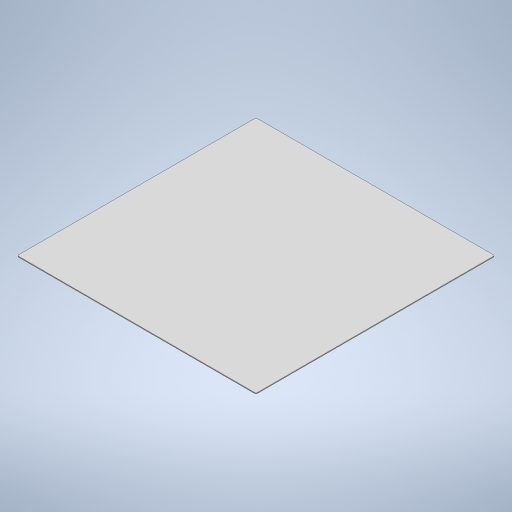
# Autodesk Inventor part: Glass top X1
Saved by Autodesk Inventor 2023 (Build 270158000, 158)
## iProperties
Created: 2022-11-22
Part Number: Glass top X1
Material: Generic
Document SubType Name: Modeling
Designer: surat
Density: 1 g/cm^3
Appearance: Default
Author: surat
Autodesk Inventor part; units mm, degrees
ref_plane "YZ Plane" through (0, 0, 0) normal (1, 0, 0) x (0, 1, 0)
ref_plane "XZ Plane" through (0, 0, 0) normal (0, 1, 0) x (-1, 0, 0)
ref_plane "XY Plane" through (0, 0, 0) normal (0, 0, 1) x (1, 0, 0)
sketch "Sketch1" plane through (0, 0, 0) normal (0, 1, 0) x (-1, 0, 0)
  line L0 (6.35, 0) -> (1365.25, 0)
  line L1 (1371.6, -6.35) -> (1371.6, -1365.25)
  line L2 (1365.25, -1371.6) -> (6.35, -1371.6)
  line L3 (0, -1365.25) -> (0, -6.35)
  line L4 (1346.2, -1346.2) -> (1346.2, -25.4)
  line L5 (1346.2, -25.4) -> (25.4, -25.4)
  line L6 (25.4, -25.4) -> (25.4, -1346.2)
  line L7 (25.4, -1346.2) -> (1346.2, -1346.2)
  line L8 (1320.8, -50.8) -> (1320.8, -1320.8)
  line L9 (1320.8, -1320.8) -> (50.8, -1320.8)
  line L10 (50.8, -1320.8) -> (50.8, -50.8)
  line L11 (50.8, -50.8) -> (1320.8, -50.8)
  line L12 (1320.8, -50.8) -> (1346.2, -25.4)
  line L13 (1320.8, -1320.8) -> (1346.2, -1346.2)
  line L14 (50.8, -1320.8) -> (25.4, -1346.2)
  line L15 (50.8, -50.8) -> (25.4, -25.4)
  line L16 (1219.2, -482.6) -> (1016, -482.6)
  line L17 (1016, -482.6) -> (1016, -889)
  line L18 (1016, -889) -> (1219.2, -889)
  line L19 (1219.2, -889) -> (1219.2, -482.6)
  line L20 (355.6, -482.6) -> (152.4, -482.6)
  line L21 (152.4, -482.6) -> (152.4, -889)
  line L22 (152.4, -889) -> (355.6, -889)
  line L23 (355.6, -889) -> (355.6, -482.6)
  line L24 (889, -1016) -> (482.6, -1016)
  line L25 (482.6, -1016) -> (482.6, -1219.2)
  line L26 (482.6, -1219.2) -> (889, -1219.2)
  line L27 (889, -1219.2) -> (889, -1016)
  line L28 (889, -152.4) -> (482.6, -152.4)
  line L29 (482.6, -152.4) -> (482.6, -355.6)
  line L30 (482.6, -355.6) -> (889, -355.6)
  line L31 (889, -355.6) -> (889, -152.4)
  circle A0 centre (685.8, -685.8) radius 254
  line L32 (889, -127) -> (482.6, -127)
  line L33 (457.2, -127) -> (457.2, -381)
  line L34 (457.2, -381) -> (914.4, -381)
  line L35 (914.4, -381) -> (914.4, -127)
  line L36 (1244.6, -457.2) -> (990.6, -457.2)
  line L37 (990.6, -457.2) -> (990.6, -914.4)
  line L38 (990.6, -914.4) -> (1244.6, -914.4)
  line L39 (1244.6, -889) -> (1244.6, -482.6)
  line L40 (914.4, -990.6) -> (457.2, -990.6)
  line L41 (457.2, -990.6) -> (457.2, -1244.6)
  line L42 (482.6, -1244.6) -> (889, -1244.6)
  line L43 (914.4, -1244.6) -> (914.4, -990.6)
  line L44 (381, -457.2) -> (127, -457.2)
  line L45 (127, -482.6) -> (127, -889)
  line L46 (127, -914.4) -> (381, -914.4)
  line L47 (381, -914.4) -> (381, -457.2)
  line L48 (152.4, -482.6) -> (50.8, -482.6)
  line L49 (127, -457.2) -> (50.8, -457.2)
  line L50 (152.4, -889) -> (50.8, -889)
  line L51 (127, -914.4) -> (50.8, -914.4)
  line L52 (355.6, -889) -> (381, -889)
  line L53 (355.6, -482.6) -> (381, -482.6)
  line L54 (457.2, -1244.6) -> (457.2, -1320.8)
  line L55 (482.6, -1219.2) -> (482.6, -1320.8)
  line L56 (889, -1219.2) -> (889, -1320.8)
  line L57 (914.4, -1244.6) -> (914.4, -1320.8)
  line L58 (1244.6, -914.4) -> (1320.8, -914.4)
  line L59 (1219.2, -889) -> (1320.8, -889)
  line L60 (1219.2, -482.6) -> (1320.8, -482.6)
  line L61 (1244.6, -457.2) -> (1320.8, -457.2)
  line L62 (889, -152.4) -> (889, -50.8)
  line L63 (914.4, -127) -> (914.4, -50.8)
  line L64 (482.6, -152.4) -> (482.6, -50.8)
  line L65 (457.2, -127) -> (457.2, -50.8)
  line L66 (889, -1016) -> (889, -990.6)
  line L67 (482.6, -1016) -> (482.6, -990.6)
  line L68 (1016, -889) -> (990.6, -889)
  line L69 (1016, -482.6) -> (990.6, -482.6)
  line L70 (889, -355.6) -> (889, -381)
  line L71 (482.6, -355.6) -> (482.6, -381)
  line L72 (914.4, -381) -> (990.6, -457.2)
  line L73 (990.6, -482.6) -> (889, -381)
  line L74 (990.6, -914.4) -> (914.4, -990.6)
  line L75 (889, -990.6) -> (990.6, -889)
  line L76 (381, -914.4) -> (457.2, -990.6)
  line L77 (482.6, -990.6) -> (381, -889)
  line L78 (457.2, -381) -> (381, -457.2)
  line L79 (482.6, -381) -> (381, -482.6)
  line L80 (1257.3, -50.8) -> (1320.8, -114.3)
  line L81 (1320.8, -1257.3) -> (1257.3, -1320.8)
  line L82 (50.8, -1257.3) -> (114.3, -1320.8)
  line L83 (50.8, -114.3) -> (114.3, -50.8)
  line L84 (68.7605, -132.2605) -> (132.2605, -68.7605)
  line L85 (68.7605, -1239.3395) -> (132.2605, -1302.8395)
  line L86 (1302.8395, -1239.3395) -> (1239.3395, -1302.8395)
  line L87 (1239.3395, -68.7605) -> (1302.8395, -132.2605)
  line L88 (1302.8395, -132.2605) -> (1320.8, -150.221)
  line L89 (1239.3395, -68.7605) -> (1221.379, -50.8)
  line L90 (1302.8395, -1239.3395) -> (1320.8, -1221.379)
  line L91 (1239.3395, -1302.8395) -> (1221.379, -1320.8)
  line L92 (132.2605, -1302.8395) -> (150.221, -1320.8)
  line L93 (68.7605, -1239.3395) -> (50.8, -1221.379)
  line L94 (132.2605, -68.7605) -> (150.221, -50.8)
  line L95 (68.7605, -132.2605) -> (50.8, -150.221)
  line L96 (1365.25, 0) -> (1371.6, -6.35)
  line L97 (1371.6, -1365.25) -> (1365.25, -1371.6)
  line L98 (6.35, -1371.6) -> (0, -1365.25)
  line L99 (6.35, 0) -> (0, -6.35)
  point P0 (0, 0)
  point P1 (1371.6, -1371.6)
  point P2 (1371.6, 0)
  point P3 (0, -1371.6)
  dimension "d0" = 1371.6
  dimension "d1" = 1371.6
  dimension "d2" = 25.4
  dimension "d3" = 25.4
  dimension "d4" = 203.2
  dimension "d5" = 406.4
  dimension "d6" = 203.2
  dimension "d7" = 406.4
  dimension "d8" = 406.4
  dimension "d9" = 203.2
  dimension "d10" = 406.4
  dimension "d11" = 203.2
  dimension "d12" = 101.6
  dimension "d13" = 101.6
  dimension "d14" = 101.6
  dimension "d15" = 101.6
  dimension "d16" = 431.8
  dimension "d17" = 431.8
  dimension "d18" = 431.8
  dimension "d19" = 431.8
  dimension "d20" = 508
  dimension "d21" = 25.4
  dimension "d22" = 25.4
  dimension "d23" = 25.4
  dimension "d24" = 25.4
  dimension "d25" = 45
  dimension "d26" = 63.5
  dimension "d27" = 45
  dimension "d28" = 45
  dimension "d29" = 45
  dimension "d30" = 25.4
  dimension "d31" = 25.4
  dimension "d32" = 25.4
  dimension "d33" = 25.4
  dimension "d34" = 6.35
  dimension "d35" = 6.35
  dimension "d36" = 6.35
  dimension "d37" = 6.35
  dimension "d38" = 6.35
  dimension "d39" = 6.35
  dimension "d40" = 6.35
  dimension "d41" = 6.35
  constraints: 192 end point, 37 point on line, 29 perpendicular, 24 parallel, 12 horizontal, 3 vertical, 1 centre point, 53 other
  measures "d0" distance of point (1371.6, -1371.6) point (0, -1371.6)
  measures "d1" distance of point (1371.6, 0) point (1371.6, -1371.6)
  measures "d2" distance between parallel lines of L1 L4
  measures "d4" distance of L18.end L17.end
  measures "d5" distance of L17.end L16.end
  measures "d6" distance of L22.end L21.end
  measures "d7" distance of L21.end L20.end
  measures "d8" distance of L26.end L25.end
  measures "d9" distance of L25.end L24.end
  measures "d10" distance of L30.end L29.end
  measures "d11" distance of L29.end L28.end
  measures "d20" diameter of A0
  measures "d21" distance between parallel lines of L31 L35
  measures "d22" distance between parallel lines of L19 L39
  measures "d23" distance between parallel lines of L27 L43
  measures "d24" distance between parallel lines of L23 L47
  measures "d25" angle to the sketch x axis of L80
  measures "d26" horizontal distance of L80.start L80.end
  measures "d27" angle to the sketch x axis of L81
  measures "d28" angle to the sketch x axis of L83
  measures "d29" angle to the sketch x axis of L82
  measures "d30" distance between parallel lines of L83 L84
  measures "d31" distance between parallel lines of L82 L85
  measures "d32" distance between parallel lines of L81 L86
  measures "d33" distance between parallel lines of L80 L87
  measures "d34" distance of L0.end point (1371.6, 0)
  measures "d35" distance of L1.start point (1371.6, 0)
  measures "d36" distance of L1.end point (1371.6, -1371.6)
  measures "d37" distance of L2.start point (1371.6, -1371.6)
  measures "d38" distance of L2.end point (0, -1371.6)
  measures "d39" distance of L3.start point (0, -1371.6)
  measures "d40" distance of L0.start point (0, 0)
  measures "d41" distance of L3.end point (0, 0)
extrude "Extrusion1" add sketch "Sketch1" along normal blind 5.08 contours L0 L96 L1 L97 L2 L98 L3 L99 | L13 L8 L12 L4 | L7 L14 L9 L13 | L12 L11 L15 L5 | L6 L15 L10 L14 | L9 L81 L8 | L8 L80 L11 | L10 L82 L9 | L81 L9 L91 L86 L90 L8 | L11 L83 L10 | L8 L88 L87 L89 L11 L80 | L82 L10 L93 L85 L92 L9 | L90 L86 L91 L9 L57 L43 L74 L38 L58 L8 | L83 L11 L94 L84 L95 L10 | L8 L61 L36 L72 L35 L63 L11 L89 L87 L88 | L92 L85 L93 L10 L51 L46 L76 L41 L54 L9 | L58 L38 L37 L68 L18 L59 L8 | L9 L56 L27 L66 L40 L43 L57 | L95 L84 L94 L11 L65 L33 L78 L44 L49 L10 | L8 L60 L16 L69 L37 L36 L61 | L63 L35 L34 L70 L31 L62 L11 | L54 L41 L40 L67 L25 L55 L9 | L10 L50 L22 L52 L47 L46 L51 | L59 L39 L60 L8 | L9 L55 L42 L56 | L49 L44 L47 L53 L20 L48 L10 | L11 L64 L29 L71 L34 L33 L65 | L62 L32 L64 L11 | L10 L48 L45 L50 | L59 L19 L60 L39 | L74 L40 L75 L37 | L42 L55 L26 L56 | L37 L73 L34 L72 | L62 L28 L64 L32 | L76 L47 L77 L40 | L45 L48 L21 L50 | L18 L17 L16 L19 | L75 L40 L77 L47 L79 L34 L73 L37 | L37 L69 L17 L68 | L26 L25 L24 L27 | L66 L24 L67 L40 | L78 L34 L79 L47 | L31 L30 L29 L28 | L34 L71 L30 L70 | L21 L20 L23 L22 | L52 L23 L53 L47 | A0
chamfer "Chamfer1" distance 1.524 angle 45 8 edges at (-1371.6, 5.08, -685.8) (-1371.6, 0, -685.8) (-685.8, 5.08, 0) (-685.8, 0, 0) (-685.8, 5.08, -1371.6) (-685.8, 0, -1371.6) (0, 5.08, -685.8) (0, 0, -685.8)
equation "\"d35\" = d34"
equation "\"d36\" = d34"
equation "\"d37\" = d36"
equation "\"d38\" = d34"
equation "\"d39\" = d38"
equation "\"d40\" = d34"
equation "\"d41\" = d40"
body "Solid1"
